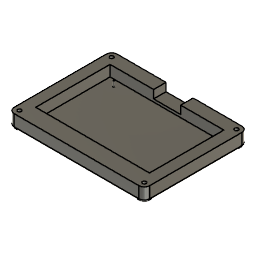
Macro bottom (Autodesk Fusion 360 design; units mm, degrees)
Autodesk Fusion 360 part; units mm, degrees
sketch "Sketch1" plane through (0, 0, 0) normal (0, 0, 1) x (1, 0, 0)
  line L0 (-135, 128.4755) -> (-30.225, 128.4755)
  line L1 (-30.225, 128.4755) -> (-30.225, 60.0051)
  line L2 (-30.225, 60.0051) -> (-135, 60.0051)
  line L3 (-135, 60.0051) -> (-135, 128.4755)
  circle A0 centre (-34.9919, 122.4579) radius 0.7
  circle A1 centre (-125.5089, 122.4579) radius 0.7
  circle A2 centre (-140, 135) radius 3
  circle A3 centre (-25, 135) radius 3
  circle A4 centre (-25, 50) radius 3
  circle A5 centre (-140, 50) radius 3
  line L4 (-145, 140) -> (-20, 140)
  line L5 (-20, 140) -> (-20, 45)
  line L6 (-20, 45) -> (-145, 45)
  line L7 (-145, 45) -> (-145, 140)
  circle A6 centre (-25, 135) radius 1.7
  circle A7 centre (-140, 135) radius 1.7
  circle A8 centre (-140, 50) radius 1.7
  circle A9 centre (-25, 50) radius 1.7
  dimension "d1" = 104.775
  dimension "d2" = 68.4704
  dimension "d17" = 1.4
  dimension "d18" = 1.4
  dimension "d24" = 6
  dimension "d25" = 6
  dimension "d26" = 6
  dimension "d28" = 6
  dimension "d29" = 3.4
  dimension "d30" = 3.4
  dimension "d31" = 3.4
  dimension "d32" = 3.4
  constraint horizontal L0
  constraint vertical L1
  constraint horizontal L2
  constraint vertical L3
  constraint horizontal L4
  constraint vertical L5
  constraint horizontal L6
  constraint vertical L7
  constraint concentric A3 A6
  constraint concentric A2 A7
  constraint concentric A5 A8
  constraint concentric A4 A9
  measures "d1" distance of L0.start L0.end
  measures "d2" distance of L0.start L2.end
  measures "d17" diameter of A0
  measures "d18" diameter of A1
  measures "d24" diameter of A2
  measures "d25" diameter of A3
  measures "d26" diameter of A4
  measures "d28" diameter of A5
  measures "d29" diameter of A6
  measures "d30" diameter of A7
  measures "d31" diameter of A8
  measures "d32" diameter of A9
extrude "Extrude1" add sketch "Sketch1" along normal blind 9.9 from surface at 3.1 contours A2 | A3 | A4 | A5 makes body 1 at (-22.2356, 136.1653, 9.7) makes body 2 at (-137.2356, 136.1653, 9.7) makes body 3 at (-22.0037, 49.8505, 9.7) makes body 4 at (-139.1875, 52.8879, 9.7)
extrude "Extrude2" add sketch "Sketch1" along normal blind 13 contours L4 L5 L6 L7 bodies 1 2 3 4
extrude "Extrude3" add sketch "Sketch1" along normal blind 3 contours L0 L1 L2 L3 bodies 1
extrude "Extrude4" add sketch "Sketch1" along normal blind 8 contours A0 | A1 bodies 1
sketch "Sketch2" plane through (0, 0, 13) normal (0, 0, 1) x (-1, 0, 0)
  circle A0 centre (25, -135) radius 1.7
  circle A1 centre (140, -50) radius 1.7
  line L0 (30.225, -60.0051) -> (135, -60.0051)
  line L1 (135, -60.0051) -> (135, -128.4755)
  line L2 (135, -128.4755) -> (30.225, -128.4755)
  line L3 (30.225, -128.4755) -> (30.225, -60.0051)
  line L4 (145, -45) -> (20, -45)
  line L5 (20, -45) -> (20, -140)
  line L6 (20, -140) -> (145, -140)
  line L7 (145, -140) -> (145, -45)
  circle A2 centre (140, -135) radius 1.7
  circle A3 centre (25, -50) radius 1.7
  line L8 (94.9004, -128.4755) -> (94.9004, -140)
  line L9 (70, -140) -> (70, -128.4755)
  constraint coincident L2 L8.start
  constraint coincident L6 L8.end
  constraint perpendicular L6 L8
  constraint coincident L6 L9.start
  constraint coincident L2 L9.end
  constraint perpendicular L2 L9
extrude "Extrude5" cut sketch "Sketch2" against normal blind 7.5 contours L2 L6 L8 L9 bodies 1
fillet "Fillet1" radius 5 4 edges at (-145, 45, 6.5) (-145, 140, 6.5) (-20, 140, 6.5) (-20, 45, 6.5) on bodies 1
fillet "Fillet2" radius 2.5 8 edges at (-143.5355, 138.5355, 0) (-82.5, 140, 0) (-21.4645, 138.5355, 0) (-20, 92.5, 0) (-21.4645, 46.4645, 0) (-82.5, 45, 0) (-143.5355, 46.4645, 0) (-145, 92.5, 0) on bodies 1
extrude "Extrude6" add sketch "Sketch1" along normal blind 2 contours A2 | A3 | A4 | A5 | A6 | A7 | A8 | A9 bodies 1
extrude "Extrude7" cut sketch "Sketch1" along normal blind 1 contours A2 | A3 | A4 | A5 | A6 | A7 | A8 | A9 bodies 1
